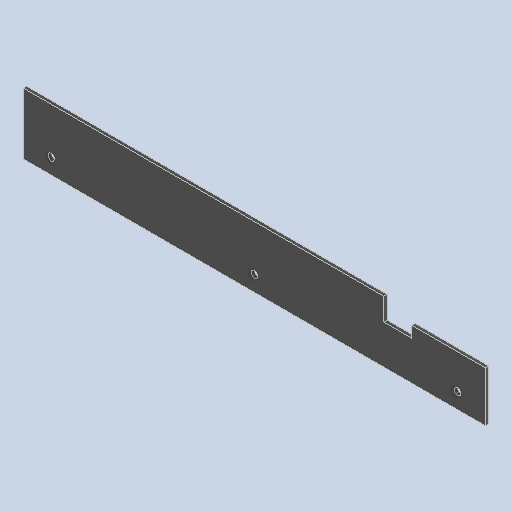
# Autodesk Inventor part: HCMUTE-CDT23-KXL_A01
Saved by Autodesk Inventor 2023 (Build 270158000, 158)
## iProperties
Created: 2023-11-20
Part Number: HCMUTE-CDT23-KXL_A01
Material: PMMA Plastic
Document SubType Name: Modeling
Designer: havie
Density: 1.188 g/cm^3
Appearance: Dark Gray
Author: havie
Autodesk Inventor part; units mm, degrees
ref_plane "YZ Plane" through (0, 0, 0) normal (1, 0, 0) x (0, 1, 0)
ref_plane "XZ Plane" through (0, 0, 0) normal (0, 1, 0) x (-1, 0, 0)
ref_plane "XY Plane" through (0, 0, 0) normal (0, 0, 1) x (1, 0, 0)
sketch "Sketch1" plane through (0, 0, 0) normal (0, 0, 1) x (1, 0, 0)
  line L0 (-207, 22.5) -> (207, 22.5)
  line L1 (207, 22.5) -> (207, -22.5)
  line L2 (207, -22.5) -> (-207, -22.5)
  line L3 (-207, -22.5) -> (-207, 22.5)
  line L4 (-207, 22.5) -> (207, -22.5) construction
  line L5 (207, 22.5) -> (-207, -22.5) construction
  point P0 (0, 0)
  dimension "d0" = 414
  dimension "d1" = 45
  constraints: 12 end point, 2 midpoint, 2 parallel, 1 horizontal, 1 perpendicular
  measures "d0" distance of L1.end L2.end
  measures "d1" distance of L2.end L0.start
extrude "Extrusion1" add sketch "Sketch1" along normal mid plane 3
sketch "Sketch2" plane through (0, 0, 1.5) normal (0, 0, 1) x (1, 0, 0)
  line L0 (-207, 22.5) -> (-207, -22.5) projected
  line L1 (207, -22.5) -> (207, 22.5) projected
  line L2 (-207, -22.5) -> (207, -22.5) projected
  point P0 (0, 0)
  point P1 (-182, -8.5)
  point P2 (0, -8.5)
  point P3 (182, -8.5)
  dimension "d4" = 25
  dimension "d5" = 25
  dimension "d6" = 182
  dimension "d7" = 14
  constraints: 2 horizontal alignment
  measures "d4" distance from line of L0 point (-182, -8.5)
  measures "d5" distance from line of L1 point (182, -8.5)
  measures "d6" distance of point (182, -8.5) point (0, -8.5)
  measures "d7" distance from line of L2 point (-182, -8.5)
hole "Hole1" at (-182, -8.5, 1.5) at (0, -8.5, 1.5) at (182, -8.5, 1.5) direction (0, 0, -1) diameter 6 depth 14.2 tip angle 118
sketch "Sketch3" plane through (0, 0, 1.5) normal (0, 0, 1) x (1, 0, 0)
  line L0 (-207, 22.5) -> (207, 22.5) projected
  line L1 (116, 22.5) -> (141, 22.5)
  line L2 (141, 22.5) -> (141, 12.5)
  line L3 (141, 12.5) -> (116, 12.5)
  line L4 (116, 12.5) -> (116, 22.5)
  line L5 (207, -22.5) -> (207, 22.5) projected
  point P0 (0, 0)
  dimension "d15" = 66
  dimension "d16" = 25
  dimension "d17" = 10
  constraints: 8 end point, 2 parallel, 1 horizontal, 1 perpendicular, 1 point on line
  measures "d15" distance between parallel lines of L5 L2
  measures "d16" distance of L2.end L3.end
  measures "d17" distance between parallel lines of L0 L3
extrude "Extrusion2" cut sketch "Sketch3" against normal blind 3
sketch "Sketch4" plane through (0, 0, 1.5) normal (0, 0, 1) x (1, 0, 0)
  line L0 (116, 22.5) -> (-207, 22.5) projected
  line L1 (-207, 22.5) -> (116, 22.5)
  line L2 (116, 22.5) -> (116, 32.5)
  line L3 (116, 32.5) -> (-207, 32.5)
  line L4 (-207, 32.5) -> (-207, 22.5)
  point P0 (0, 0)
  dimension "d20" = 10
  constraints: 8 end point, 2 parallel, 1 horizontal, 1 perpendicular, 1 vertical alignment
  measures "d20" distance of L3.end L0.end
extrude "Extrusion3" add sketch "Sketch4" against normal blind 3
equation "\"d5\" = d4"
body "Solid1"
